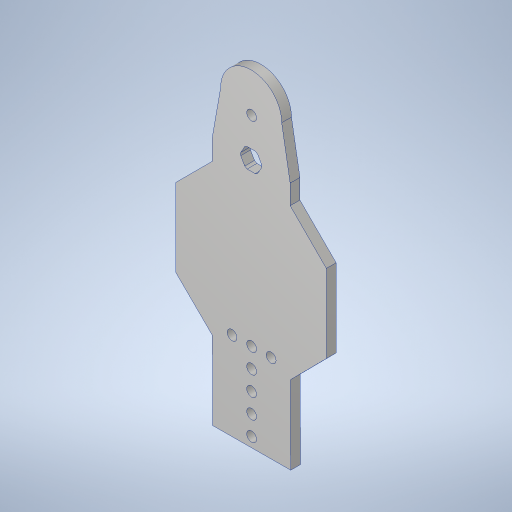
# Autodesk Inventor part: CL1-001
Saved by Autodesk Inventor 2023.4 (Build 274418000, 418)
## iProperties
Created: 2025-01-17
Part Number: CL1-001
Material: Aluminum 6061
Document SubType Name: Modeling
Designer: mavericks
Density: 2.7 g/cm^3
Appearance: Aluminum - Flat
Author: mavericks
Autodesk Inventor part; units mm, degrees
ref_plane "YZ Plane" through (0, 0, 0) normal (1, 0, 0) x (0, 1, 0)
ref_plane "XZ Plane" through (0, 0, 0) normal (0, 1, 0) x (-1, 0, 0)
ref_plane "XY Plane" through (0, 0, 0) normal (0, 0, 1) x (1, 0, 0)
sketch "Sketch1" plane through (0, 0, 0) normal (0, 0, 1) x (1, 0, 0)
  line L0 (-25.5248, 25.2745) -> (-25.2745, -25.5248) construction
  line L1 (-25.2745, -25.5248) -> (25.5248, -25.2745) construction
  line L2 (25.5248, -25.2745) -> (25.2745, 25.5248) construction
  line L3 (25.2745, 25.5248) -> (-25.2745, -25.5248) construction
  line L4 (-25.5248, 25.2745) -> (25.5248, -25.2745) construction
  line L5 (25.2745, 25.5248) -> (48.7045, 49.1868) construction
  line L6 (-25.5248, 25.2745) -> (-49.1868, 48.7045) construction
  line L7 (48.7045, 49.1868) -> (48.7045, 99.9868) construction
  line L8 (-49.1868, 48.7045) -> (-49.1868, 99.5045) construction
  line L9 (-49.1868, 99.5045) -> (-25.6406, 123.0507) construction
  line L10 (48.7045, 99.9868) -> (25.1582, 123.533) construction
  line L11 (-25.6406, 123.0507) -> (-25.6406, 135.7507) construction
  line L12 (25.1582, 123.533) -> (25.1582, 136.233) construction
  line L13 (25.1582, 136.233) -> (19.6449, 167.5007) construction
  line L14 (-25.6406, 135.7507) -> (-20.0422, 167.5007) construction
  line L15 (-20.0422, 167.5007) -> (19.6449, 167.5007) construction
  arc A0 (19.6449, 167.5007) -> (-20.0422, 167.5007) centre (-0.1987, 167.5007) ccw construction
  line L16 (-25.2745, -25.5248) -> (25.5248, -25.2745)
  line L17 (25.5248, -25.2745) -> (25.2745, 25.5248)
  line L18 (48.7045, 49.1868) -> (25.2745, 25.5248)
  line L19 (48.7045, 49.1868) -> (48.7045, 99.9868)
  line L20 (48.7045, 99.9868) -> (25.1582, 123.533)
  line L21 (25.1582, 123.533) -> (25.1582, 136.233)
  line L22 (25.1582, 136.233) -> (19.6449, 167.5007)
  line L23 (-20.0422, 167.5007) -> (-25.6406, 135.7507)
  line L24 (-25.6406, 135.7507) -> (-25.6406, 123.0507)
  line L25 (-25.6406, 123.0507) -> (-49.1868, 99.5045)
  line L26 (-49.1868, 99.5045) -> (-49.1868, 48.7045)
  line L27 (-49.1868, 48.7045) -> (-25.5248, 25.2745)
  line L28 (-25.5248, 25.2745) -> (-25.2745, -25.5248)
  arc A1 (19.6449, 167.5007) -> (-20.0422, 167.5007) centre (-0.1987, 167.5007) ccw
  point P0 (0, 0)
  dimension "d0" = 50.8
  dimension "d1" = 50.8
  dimension "d2" = 33.2994
  dimension "d3" = 33.2994
  dimension "d4" = 135
  dimension "d5" = 135
  dimension "d6" = 50.8
  dimension "d7" = 50.8
  dimension "d8" = 33.2994
  dimension "d9" = 33.2994
  dimension "d10" = 135
  dimension "d11" = 135
  dimension "d12" = 12.7
  dimension "d13" = 12.7
  dimension "d15" = 31.75
  dimension "d16" = 170
  dimension "d17" = 31.75
  dimension "d18" = 170
  constraints: 58 end point, 11 equal length, 4 point on circle, 4 vertical, 3 midpoint, 2 centre point, 2 perpendicular, 1 coincident, 1 horizontal
  measures "d0" distance of L1.end L0.end
  measures "d1" distance of L0.end L0.start
  measures "d2" distance of L2.end L5.end
  measures "d3" distance of L0.start L6.end
  measures "d4" angle of L2 L5
  measures "d5" angle of L0 L6
  measures "d6" distance of L5.end L7.end
  measures "d7" distance of L6.end L8.end
  measures "d8" distance of L8.end L9.end
  measures "d9" distance of L7.end L10.end
  measures "d10" angle of L10 L7
  measures "d11" angle of L9 L8
  measures "d12" distance of L9.end L11.end
  measures "d13" distance of L10.end L12.end
  measures "d15" distance of L12.end L13.end
  measures "d16" angle of L13 L12
  measures "d17" vertical distance of L11.end L14.end
  measures "d18" angle of L11 L14
extrude "Extrusion1" add sketch "Sketch1" along normal blind 6.35
sketch "Sketch2" plane through (0, 0, 0) normal (0, 0, -1) x (-1, 0, 0)
  line L0 (25.2745, -25.5248) -> (-25.5248, -25.2745) projected
  line L1 (-25.5248, -25.2745) -> (-25.2745, 25.5248) projected
  arc A0 (20.0422, 167.5007) -> (-19.6449, 167.5007) centre (0.1987, 167.5007) ccw projected
  line L2 (3.8648, 142.8942) -> (7.531, 136.5442)
  line L3 (7.531, 136.5442) -> (3.8648, 130.1942)
  line L4 (3.8648, 130.1942) -> (-3.4675, 130.1942)
  line L5 (-3.4675, 130.1942) -> (-7.1337, 136.5442)
  line L6 (-7.1337, 136.5442) -> (-3.4675, 142.8942)
  line L7 (-3.4675, 142.8942) -> (3.8648, 142.8942)
  circle A1 centre (0.1987, 136.5442) radius 6.8707
  point P0 (0, 0)
  point P1 (-0.0939, -19.0498)
  point P2 (-0.0939, -6.3498)
  point P3 (-0.0939, 6.3502)
  point P4 (-0.0939, 19.0502)
  point P5 (-0.0939, 31.7502)
  point P6 (12.6061, 31.7502)
  point P7 (-12.7939, 31.7502)
  point P8 (-0.0939, 161.9442)
  point P9 (0.1987, 187.3442)
  point P10 (0.1987, 187.3442)
  point P11 (2.8224, 130.1942)
  point P12 (4.386, 131.097)
  point P13 (7.0098, 135.6415)
  point P14 (7.0098, 137.447)
  point P15 (4.386, 141.9915)
  point P16 (2.8224, 142.8942)
  point P17 (-2.4251, 142.8942)
  point P18 (-3.9887, 141.9915)
  point P19 (-6.6125, 137.447)
  point P20 (-6.6125, 135.6415)
  point P21 (-3.9887, 131.097)
  point P22 (-2.4251, 130.1942)
  dimension "d21" = 6.35
  dimension "d22" = 25.4
  dimension "d23" = 12.7
  dimension "d24" = 12.7
  dimension "d25" = 12.7
  dimension "d26" = 12.7
  dimension "d27" = 12.7
  dimension "d28" = 12.7
  dimension "d29" = 25.4
  dimension "d31" = 25.4
  dimension "d41" = 13.7414
  dimension "d42" = 12.7
  constraints: 12 end point, 6 vertical alignment, 2 horizontal alignment, 2 point on circle, 1 centre point, 1 coincident, 1 horizontal, 13 other
  measures "d21" distance from line of L0 point (-0.094, -19.05)
  measures "d22" distance from line of point (-0.094, -19.05) L1
  measures "d23" distance of point (-0.094, -19.05) point (-0.094, -6.35)
  measures "d24" distance of point (-0.094, 6.35) point (-0.094, -6.35)
  measures "d25" distance of point (-0.094, 6.35) point (-0.094, 19.05)
  measures "d26" distance of point (-0.094, 19.05) point (-0.094, 31.75)
  measures "d27" distance of point (-0.094, 31.75) point (-12.794, 31.75)
  measures "d28" distance of point (-0.094, 31.75) point (12.606, 31.75)
  measures "d29" vertical distance of point (0.199, 187.344) point (-0.094, 161.944)
  measures "d31" vertical distance of point (-0.094, 161.944) point (0.199, 136.544)
  measures "d41" diameter of A1
  measures "d42" distance between parallel lines of L4 L7
hole "Hole1" at (0.0939, -19.0498, 0) at (0.0939, -6.3498, 0) at (0.0939, 6.3502, 0) at (0.0939, 19.0502, 0) at (0.0939, 31.7502, 0) at (-12.6061, 31.7502, 0) at (12.7939, 31.7502, 0) at (0.0939, 161.9442, 0) direction (0, 0, 1) diameter 6.35 end through all clearance for "Flat Head Machine Screw (82)" size "1/4" standard "Ansi Unified Screw Threads"
extrude "Extrusion2" cut sketch "Sketch2" against normal blind 6.35 contours L2 A1 L3 L4 L5 L6 L7
equation "\"d3\" = d2"
equation "\"d5\" = d4"
equation "\"d7\" = d6"
equation "\"d11\" = d10"
equation "\"d13\" = d12"
equation "\"d17\" = d15"
equation "\"d18\" = d16"
equation "\"d24\" = d23"
equation "\"d25\" = d23"
equation "\"d28\" = d27"
body "Solid1"
